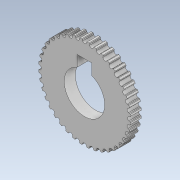
# Autodesk Inventor part: 2GT_40T
Saved by Autodesk Inventor 2022 (Build 260153000, 153)
## iProperties
Created: 2023-05-04
Part Number: 2GT_40T
Material: 一般
Document SubType Name: Modeling
Designer: Johnny Jou
Density: 1 g/cm^3
Appearance: 預設
Author: Johnny Jou
Autodesk Inventor part; units mm, degrees
ref_plane "YZ Plane" through (0, 0, 0) normal (1, 0, 0) x (0, 1, 0)
ref_plane "XZ Plane" through (0, 0, 0) normal (0, 1, 0) x (-1, 0, 0)
ref_plane "XY Plane" through (0, 0, 0) normal (0, 0, 1) x (1, 0, 0)
sketch "草圖1" plane through (0, 0, 0) normal (0, 0, 1) x (1, 0, 0)
  arc A0 (1.3466, 12.2657) -> (1.2112, 12.4161) centre (1.1966, 12.2668) ccw
  arc A1 (1.2112, 12.4161) -> (0.746, 12.4527) centre (0, 0) ccw
  arc A2 (0.746, 12.4527) -> (0.5887, 12.3254) centre (0.7371, 12.3029) ccw
  arc A3 (0.4989, 12.0368) -> (0.5887, 12.3254) centre (-0.4, 12.475) ccw
  arc A4 (-0.4989, 12.0368) -> (0.4989, 12.0368) centre (0, 12.28) ccw
  arc A5 (-0.5887, 12.3254) -> (-0.4989, 12.0368) centre (0.4, 12.475) ccw
  arc A6 (-0.5887, 12.3254) -> (-0.746, 12.4527) centre (-0.7371, 12.3029) ccw
  arc A7 (-0.746, 12.4527) -> (-1.2112, 12.4161) centre (0, 0) ccw
  arc A8 (-1.2112, 12.4161) -> (-1.3466, 12.2657) centre (-1.1966, 12.2668) ccw
  arc A9 (-1.3902, 11.9666) -> (-1.3466, 12.2657) centre (-2.3466, 12.2588) ccw
  arc A10 (-2.3757, 11.8106) -> (-1.3902, 11.9666) centre (-1.921, 12.1288) ccw
  arc A11 (-2.5096, 12.0815) -> (-2.3757, 11.8106) centre (-1.5564, 12.384) ccw
  arc A12 (-2.5096, 12.0815) -> (-2.6849, 12.1827) centre (-2.6526, 12.0362) ccw
  arc A13 (-2.6849, 12.1827) -> (-3.1386, 12.0737) centre (0, 0) ccw
  arc A14 (-3.1386, 12.0737) -> (-3.2488, 11.9041) centre (-3.1008, 11.9286) ccw
  arc A15 (-3.2451, 11.6018) -> (-3.2488, 11.9041) centre (-4.2354, 11.7408) ccw
  arc A16 (-4.194, 11.2935) -> (-3.2451, 11.6018) centre (-3.7947, 11.679) ccw
  arc A17 (-4.3687, 11.5402) -> (-4.194, 11.2935) centre (-3.4746, 11.988) ccw
  arc A18 (-4.3687, 11.5402) -> (-4.5576, 11.6127) centre (-4.5028, 11.473) ccw
  arc A19 (-4.5576, 11.6127) -> (-4.9887, 11.4341) centre (0, 0) ccw
  arc A20 (-4.9887, 11.4341) -> (-5.071, 11.2493) centre (-4.9287, 11.2966) ccw
  arc A21 (-5.0201, 10.9514) -> (-5.071, 11.2493) centre (-6.0199, 10.9337) ccw
  arc A22 (-5.9091, 10.4984) -> (-5.0201, 10.9514) centre (-5.575, 10.9416) ccw
  arc A23 (-6.1202, 10.7147) -> (-5.9091, 10.4984) centre (-5.3071, 11.2969) ccw
  arc A24 (-6.1202, 10.7147) -> (-6.3181, 10.7567) centre (-6.2421, 10.6274) ccw
  arc A25 (-6.3181, 10.7567) -> (-6.7159, 10.5129) centre (0, 0) ccw
  arc A26 (-6.7159, 10.5129) -> (-6.7684, 10.3175) centre (-6.6352, 10.3865) ccw
  arc A27 (-6.6715, 10.0312) -> (-6.7684, 10.3175) centre (-7.6562, 9.8574) ccw
  arc A28 (-7.4787, 9.4447) -> (-6.6715, 10.0312) centre (-7.218, 9.9347) ccw
  arc A29 (-7.721, 9.6254) -> (-7.4787, 9.4447) centre (-7.009, 10.3276) ccw
  arc A30 (-7.721, 9.6254) -> (-7.923, 9.6359) centre (-7.8278, 9.5201) ccw
  arc A31 (-7.923, 9.6359) -> (-8.2778, 9.3329) centre (0, 0) ccw
  arc A32 (-8.2778, 9.3329) -> (-8.2991, 9.1317) centre (-8.1783, 9.2207) ccw
  arc A33 (-8.1585, 8.8641) -> (-8.2991, 9.1317) centre (-9.104, 8.5383) ccw
  arc A34 (-8.8641, 8.1585) -> (-8.1585, 8.8641) centre (-8.6833, 8.6833) ccw
  arc A35 (-9.1317, 8.2991) -> (-8.8641, 8.1585) centre (-8.5383, 9.104) ccw
  arc A36 (-9.1317, 8.2991) -> (-9.3329, 8.2778) centre (-9.2207, 8.1783) ccw
  arc A37 (-9.3329, 8.2778) -> (-9.6359, 7.923) centre (0, 0) ccw
  arc A38 (-9.6359, 7.923) -> (-9.6254, 7.721) centre (-9.5201, 7.8278) ccw
  arc A39 (-9.4447, 7.4787) -> (-9.6254, 7.721) centre (-10.3276, 7.009) ccw
  arc A40 (-10.0312, 6.6715) -> (-9.4447, 7.4787) centre (-9.9347, 7.218) ccw
  arc A41 (-10.3175, 6.7684) -> (-10.0312, 6.6715) centre (-9.8574, 7.6562) ccw
  arc A42 (-10.3175, 6.7684) -> (-10.5129, 6.7159) centre (-10.3865, 6.6352) ccw
  arc A43 (-10.5129, 6.7159) -> (-10.7567, 6.3181) centre (0, 0) ccw
  arc A44 (-10.7567, 6.3181) -> (-10.7147, 6.1202) centre (-10.6274, 6.2421) ccw
  arc A45 (-10.4984, 5.9091) -> (-10.7147, 6.1202) centre (-11.2969, 5.3071) ccw
  arc A46 (-10.9514, 5.0201) -> (-10.4984, 5.9091) centre (-10.9416, 5.575) ccw
  arc A47 (-11.2493, 5.071) -> (-10.9514, 5.0201) centre (-10.9337, 6.0199) ccw
  arc A48 (-11.2493, 5.071) -> (-11.4341, 4.9887) centre (-11.2966, 4.9287) ccw
  arc A49 (-11.4341, 4.9887) -> (-11.6127, 4.5576) centre (0, 0) ccw
  arc A50 (-11.6127, 4.5576) -> (-11.5402, 4.3687) centre (-11.473, 4.5028) ccw
  arc A51 (-11.2935, 4.194) -> (-11.5402, 4.3687) centre (-11.988, 3.4746) ccw
  arc A52 (-11.6018, 3.2451) -> (-11.2935, 4.194) centre (-11.679, 3.7947) ccw
  arc A53 (-11.9041, 3.2488) -> (-11.6018, 3.2451) centre (-11.7408, 4.2354) ccw
  arc A54 (-11.9041, 3.2488) -> (-12.0737, 3.1386) centre (-11.9286, 3.1008) ccw
  arc A55 (-12.0737, 3.1386) -> (-12.1827, 2.6849) centre (0, 0) ccw
  arc A56 (-12.1827, 2.6849) -> (-12.0815, 2.5096) centre (-12.0362, 2.6526) ccw
  arc A57 (-11.8106, 2.3757) -> (-12.0815, 2.5096) centre (-12.384, 1.5564) ccw
  arc A58 (-11.9666, 1.3902) -> (-11.8106, 2.3757) centre (-12.1288, 1.921) ccw
  arc A59 (-12.2657, 1.3466) -> (-11.9666, 1.3902) centre (-12.2588, 2.3466) ccw
  arc A60 (-12.2657, 1.3466) -> (-12.4161, 1.2112) centre (-12.2668, 1.1966) ccw
  arc A61 (-12.4161, 1.2112) -> (-12.4527, 0.746) centre (0, 0) ccw
  arc A62 (-12.4527, 0.746) -> (-12.3254, 0.5887) centre (-12.3029, 0.7371) ccw
  arc A63 (-12.0368, 0.4989) -> (-12.3254, 0.5887) centre (-12.475, -0.4) ccw
  arc A64 (-12.0368, -0.4989) -> (-12.0368, 0.4989) centre (-12.28, 0) ccw
  arc A65 (-12.3254, -0.5887) -> (-12.0368, -0.4989) centre (-12.475, 0.4) ccw
  arc A66 (-12.3254, -0.5887) -> (-12.4527, -0.746) centre (-12.3029, -0.7371) ccw
  arc A67 (-12.4527, -0.746) -> (-12.4161, -1.2112) centre (0, 0) ccw
  arc A68 (-12.4161, -1.2112) -> (-12.2657, -1.3466) centre (-12.2668, -1.1966) ccw
  arc A69 (-11.9666, -1.3902) -> (-12.2657, -1.3466) centre (-12.2588, -2.3466) ccw
  arc A70 (-11.8106, -2.3757) -> (-11.9666, -1.3902) centre (-12.1288, -1.921) ccw
  arc A71 (-12.0815, -2.5096) -> (-11.8106, -2.3757) centre (-12.384, -1.5564) ccw
  arc A72 (-12.0815, -2.5096) -> (-12.1827, -2.6849) centre (-12.0362, -2.6526) ccw
  arc A73 (-12.1827, -2.6849) -> (-12.0737, -3.1386) centre (0, 0) ccw
  arc A74 (-12.0737, -3.1386) -> (-11.9041, -3.2488) centre (-11.9286, -3.1008) ccw
  arc A75 (-11.6018, -3.2451) -> (-11.9041, -3.2488) centre (-11.7408, -4.2354) ccw
  arc A76 (-11.2935, -4.194) -> (-11.6018, -3.2451) centre (-11.679, -3.7947) ccw
  arc A77 (-11.5402, -4.3687) -> (-11.2935, -4.194) centre (-11.988, -3.4746) ccw
  arc A78 (-11.5402, -4.3687) -> (-11.6127, -4.5576) centre (-11.473, -4.5028) ccw
  arc A79 (-11.6127, -4.5576) -> (-11.4341, -4.9887) centre (0, 0) ccw
  arc A80 (-11.4341, -4.9887) -> (-11.2493, -5.071) centre (-11.2966, -4.9287) ccw
  arc A81 (-10.9514, -5.0201) -> (-11.2493, -5.071) centre (-10.9337, -6.0199) ccw
  arc A82 (-10.4984, -5.9091) -> (-10.9514, -5.0201) centre (-10.9416, -5.575) ccw
  arc A83 (-10.7147, -6.1202) -> (-10.4984, -5.9091) centre (-11.2969, -5.3071) ccw
  arc A84 (-10.7147, -6.1202) -> (-10.7567, -6.3181) centre (-10.6274, -6.2421) ccw
  arc A85 (-10.7567, -6.3181) -> (-10.5129, -6.7159) centre (0, 0) ccw
  arc A86 (-10.5129, -6.7159) -> (-10.3175, -6.7684) centre (-10.3865, -6.6352) ccw
  arc A87 (-10.0312, -6.6715) -> (-10.3175, -6.7684) centre (-9.8574, -7.6562) ccw
  arc A88 (-9.4447, -7.4787) -> (-10.0312, -6.6715) centre (-9.9347, -7.218) ccw
  arc A89 (-9.6254, -7.721) -> (-9.4447, -7.4787) centre (-10.3276, -7.009) ccw
  arc A90 (-9.6254, -7.721) -> (-9.6359, -7.923) centre (-9.5201, -7.8278) ccw
  arc A91 (-9.6359, -7.923) -> (-9.3329, -8.2778) centre (0, 0) ccw
  arc A92 (-9.3329, -8.2778) -> (-9.1317, -8.2991) centre (-9.2207, -8.1783) ccw
  arc A93 (-8.8641, -8.1585) -> (-9.1317, -8.2991) centre (-8.5383, -9.104) ccw
  arc A94 (-8.1585, -8.8641) -> (-8.8641, -8.1585) centre (-8.6833, -8.6833) ccw
  arc A95 (-8.2991, -9.1317) -> (-8.1585, -8.8641) centre (-9.104, -8.5383) ccw
  arc A96 (-8.2991, -9.1317) -> (-8.2778, -9.3329) centre (-8.1783, -9.2207) ccw
  arc A97 (-8.2778, -9.3329) -> (-7.923, -9.6359) centre (0, 0) ccw
  arc A98 (-7.923, -9.6359) -> (-7.721, -9.6254) centre (-7.8278, -9.5201) ccw
  arc A99 (-7.4787, -9.4447) -> (-7.721, -9.6254) centre (-7.009, -10.3276) ccw
  arc A100 (-6.6715, -10.0312) -> (-7.4787, -9.4447) centre (-7.218, -9.9347) ccw
  arc A101 (-6.7684, -10.3175) -> (-6.6715, -10.0312) centre (-7.6562, -9.8574) ccw
  arc A102 (-6.7684, -10.3175) -> (-6.7159, -10.5129) centre (-6.6352, -10.3865) ccw
  arc A103 (-6.7159, -10.5129) -> (-6.3181, -10.7567) centre (0, 0) ccw
  arc A104 (-6.3181, -10.7567) -> (-6.1202, -10.7147) centre (-6.2421, -10.6274) ccw
  arc A105 (-5.9091, -10.4984) -> (-6.1202, -10.7147) centre (-5.3071, -11.2969) ccw
  arc A106 (-5.0201, -10.9514) -> (-5.9091, -10.4984) centre (-5.575, -10.9416) ccw
  arc A107 (-5.071, -11.2493) -> (-5.0201, -10.9514) centre (-6.0199, -10.9337) ccw
  arc A108 (-5.071, -11.2493) -> (-4.9887, -11.4341) centre (-4.9287, -11.2966) ccw
  arc A109 (-4.9887, -11.4341) -> (-4.5576, -11.6127) centre (0, 0) ccw
  arc A110 (-4.5576, -11.6127) -> (-4.3687, -11.5402) centre (-4.5028, -11.473) ccw
  arc A111 (-4.194, -11.2935) -> (-4.3687, -11.5402) centre (-3.4746, -11.988) ccw
  arc A112 (-3.2451, -11.6018) -> (-4.194, -11.2935) centre (-3.7947, -11.679) ccw
  arc A113 (-3.2488, -11.9041) -> (-3.2451, -11.6018) centre (-4.2354, -11.7408) ccw
  arc A114 (-3.2488, -11.9041) -> (-3.1386, -12.0737) centre (-3.1008, -11.9286) ccw
  arc A115 (-3.1386, -12.0737) -> (-2.6849, -12.1827) centre (0, 0) ccw
  arc A116 (-2.6849, -12.1827) -> (-2.5096, -12.0815) centre (-2.6526, -12.0362) ccw
  arc A117 (-2.3757, -11.8106) -> (-2.5096, -12.0815) centre (-1.5564, -12.384) ccw
  arc A118 (-1.3902, -11.9666) -> (-2.3757, -11.8106) centre (-1.921, -12.1288) ccw
  arc A119 (-1.3466, -12.2657) -> (-1.3902, -11.9666) centre (-2.3466, -12.2588) ccw
  arc A120 (-1.3466, -12.2657) -> (-1.2112, -12.4161) centre (-1.1966, -12.2668) ccw
  arc A121 (-1.2112, -12.4161) -> (-0.746, -12.4527) centre (0, 0) ccw
  arc A122 (-0.746, -12.4527) -> (-0.5887, -12.3254) centre (-0.7371, -12.3029) ccw
  arc A123 (-0.4989, -12.0368) -> (-0.5887, -12.3254) centre (0.4, -12.475) ccw
  arc A124 (0.4989, -12.0368) -> (-0.4989, -12.0368) centre (0, -12.28) ccw
  arc A125 (0.5887, -12.3254) -> (0.4989, -12.0368) centre (-0.4, -12.475) ccw
  arc A126 (0.5887, -12.3254) -> (0.746, -12.4527) centre (0.7371, -12.3029) ccw
  arc A127 (0.746, -12.4527) -> (1.2112, -12.4161) centre (0, 0) ccw
  arc A128 (1.2112, -12.4161) -> (1.3466, -12.2657) centre (1.1966, -12.2668) ccw
  arc A129 (1.3902, -11.9666) -> (1.3466, -12.2657) centre (2.3466, -12.2588) ccw
  arc A130 (2.3757, -11.8106) -> (1.3902, -11.9666) centre (1.921, -12.1288) ccw
  arc A131 (2.5096, -12.0815) -> (2.3757, -11.8106) centre (1.5564, -12.384) ccw
  arc A132 (2.5096, -12.0815) -> (2.6849, -12.1827) centre (2.6526, -12.0362) ccw
  arc A133 (2.6849, -12.1827) -> (3.1386, -12.0737) centre (0, 0) ccw
  arc A134 (3.1386, -12.0737) -> (3.2488, -11.9041) centre (3.1008, -11.9286) ccw
  arc A135 (3.2451, -11.6018) -> (3.2488, -11.9041) centre (4.2354, -11.7408) ccw
  arc A136 (4.194, -11.2935) -> (3.2451, -11.6018) centre (3.7947, -11.679) ccw
  arc A137 (4.3687, -11.5402) -> (4.194, -11.2935) centre (3.4746, -11.988) ccw
  arc A138 (4.3687, -11.5402) -> (4.5576, -11.6127) centre (4.5028, -11.473) ccw
  arc A139 (4.5576, -11.6127) -> (4.9887, -11.4341) centre (0, 0) ccw
  arc A140 (4.9887, -11.4341) -> (5.071, -11.2493) centre (4.9287, -11.2966) ccw
  arc A141 (5.0201, -10.9514) -> (5.071, -11.2493) centre (6.0199, -10.9337) ccw
  arc A142 (5.9091, -10.4984) -> (5.0201, -10.9514) centre (5.575, -10.9416) ccw
  arc A143 (6.1202, -10.7147) -> (5.9091, -10.4984) centre (5.3071, -11.2969) ccw
  arc A144 (6.1202, -10.7147) -> (6.3181, -10.7567) centre (6.2421, -10.6274) ccw
  arc A145 (6.3181, -10.7567) -> (6.7159, -10.5129) centre (0, 0) ccw
  arc A146 (6.7159, -10.5129) -> (6.7684, -10.3175) centre (6.6352, -10.3865) ccw
  arc A147 (6.6715, -10.0312) -> (6.7684, -10.3175) centre (7.6562, -9.8574) ccw
  arc A148 (7.4787, -9.4447) -> (6.6715, -10.0312) centre (7.218, -9.9347) ccw
  arc A149 (7.721, -9.6254) -> (7.4787, -9.4447) centre (7.009, -10.3276) ccw
  arc A150 (7.721, -9.6254) -> (7.923, -9.6359) centre (7.8278, -9.5201) ccw
  arc A151 (7.923, -9.6359) -> (8.2778, -9.3329) centre (0, 0) ccw
  arc A152 (8.2778, -9.3329) -> (8.2991, -9.1317) centre (8.1783, -9.2207) ccw
  arc A153 (8.1585, -8.8641) -> (8.2991, -9.1317) centre (9.104, -8.5383) ccw
  arc A154 (8.8641, -8.1585) -> (8.1585, -8.8641) centre (8.6833, -8.6833) ccw
  arc A155 (9.1317, -8.2991) -> (8.8641, -8.1585) centre (8.5383, -9.104) ccw
  arc A156 (9.1317, -8.2991) -> (9.3329, -8.2778) centre (9.2207, -8.1783) ccw
  arc A157 (9.3329, -8.2778) -> (9.6359, -7.923) centre (0, 0) ccw
  arc A158 (9.6359, -7.923) -> (9.6254, -7.721) centre (9.5201, -7.8278) ccw
  arc A159 (9.4447, -7.4787) -> (9.6254, -7.721) centre (10.3276, -7.009) ccw
  arc A160 (10.0312, -6.6715) -> (9.4447, -7.4787) centre (9.9347, -7.218) ccw
  arc A161 (10.3175, -6.7684) -> (10.0312, -6.6715) centre (9.8574, -7.6562) ccw
  arc A162 (10.3175, -6.7684) -> (10.5129, -6.7159) centre (10.3865, -6.6352) ccw
  arc A163 (10.5129, -6.7159) -> (10.7567, -6.3181) centre (0, 0) ccw
  arc A164 (10.7567, -6.3181) -> (10.7147, -6.1202) centre (10.6274, -6.2421) ccw
  arc A165 (10.4984, -5.9091) -> (10.7147, -6.1202) centre (11.2969, -5.3071) ccw
  arc A166 (10.9514, -5.0201) -> (10.4984, -5.9091) centre (10.9416, -5.575) ccw
  arc A167 (11.2493, -5.071) -> (10.9514, -5.0201) centre (10.9337, -6.0199) ccw
  arc A168 (11.2493, -5.071) -> (11.4341, -4.9887) centre (11.2966, -4.9287) ccw
  arc A169 (11.4341, -4.9887) -> (11.6127, -4.5576) centre (0, 0) ccw
  arc A170 (11.6127, -4.5576) -> (11.5402, -4.3687) centre (11.473, -4.5028) ccw
  arc A171 (11.2935, -4.194) -> (11.5402, -4.3687) centre (11.988, -3.4746) ccw
  arc A172 (11.6018, -3.2451) -> (11.2935, -4.194) centre (11.679, -3.7947) ccw
  arc A173 (11.9041, -3.2488) -> (11.6018, -3.2451) centre (11.7408, -4.2354) ccw
  arc A174 (11.9041, -3.2488) -> (12.0737, -3.1386) centre (11.9286, -3.1008) ccw
  arc A175 (12.0737, -3.1386) -> (12.1827, -2.6849) centre (0, 0) ccw
  arc A176 (12.1827, -2.6849) -> (12.0815, -2.5096) centre (12.0362, -2.6526) ccw
  arc A177 (11.8106, -2.3757) -> (12.0815, -2.5096) centre (12.384, -1.5564) ccw
  arc A178 (11.9666, -1.3902) -> (11.8106, -2.3757) centre (12.1288, -1.921) ccw
  arc A179 (12.2657, -1.3466) -> (11.9666, -1.3902) centre (12.2588, -2.3466) ccw
  arc A180 (12.2657, -1.3466) -> (12.4161, -1.2112) centre (12.2668, -1.1966) ccw
  arc A181 (12.4161, -1.2112) -> (12.4527, -0.746) centre (0, 0) ccw
  arc A182 (12.4527, -0.746) -> (12.3254, -0.5887) centre (12.3029, -0.7371) ccw
  arc A183 (12.0368, -0.4989) -> (12.3254, -0.5887) centre (12.475, 0.4) ccw
  arc A184 (12.0368, 0.4989) -> (12.0368, -0.4989) centre (12.28, 0) ccw
  arc A185 (12.3254, 0.5887) -> (12.0368, 0.4989) centre (12.475, -0.4) ccw
  arc A186 (12.3254, 0.5887) -> (12.4527, 0.746) centre (12.3029, 0.7371) ccw
  arc A187 (12.4527, 0.746) -> (12.4161, 1.2112) centre (0, 0) ccw
  arc A188 (12.4161, 1.2112) -> (12.2657, 1.3466) centre (12.2668, 1.1966) ccw
  arc A189 (11.9666, 1.3902) -> (12.2657, 1.3466) centre (12.2588, 2.3466) ccw
  arc A190 (11.8106, 2.3757) -> (11.9666, 1.3902) centre (12.1288, 1.921) ccw
  arc A191 (12.0815, 2.5096) -> (11.8106, 2.3757) centre (12.384, 1.5564) ccw
  arc A192 (12.0815, 2.5096) -> (12.1827, 2.6849) centre (12.0362, 2.6526) ccw
  arc A193 (12.1827, 2.6849) -> (12.0737, 3.1386) centre (0, 0) ccw
  arc A194 (12.0737, 3.1386) -> (11.9041, 3.2488) centre (11.9286, 3.1008) ccw
  arc A195 (11.6018, 3.2451) -> (11.9041, 3.2488) centre (11.7408, 4.2354) ccw
  arc A196 (11.2935, 4.194) -> (11.6018, 3.2451) centre (11.679, 3.7947) ccw
  arc A197 (11.5402, 4.3687) -> (11.2935, 4.194) centre (11.988, 3.4746) ccw
  arc A198 (11.5402, 4.3687) -> (11.6127, 4.5576) centre (11.473, 4.5028) ccw
  arc A199 (11.6127, 4.5576) -> (11.4341, 4.9887) centre (0, 0) ccw
  arc A200 (11.4341, 4.9887) -> (11.2493, 5.071) centre (11.2966, 4.9287) ccw
  arc A201 (10.9514, 5.0201) -> (11.2493, 5.071) centre (10.9337, 6.0199) ccw
  arc A202 (10.4984, 5.9091) -> (10.9514, 5.0201) centre (10.9416, 5.575) ccw
  arc A203 (10.7147, 6.1202) -> (10.4984, 5.9091) centre (11.2969, 5.3071) ccw
  arc A204 (10.7147, 6.1202) -> (10.7567, 6.3181) centre (10.6274, 6.2421) ccw
  arc A205 (10.7567, 6.3181) -> (10.5129, 6.7159) centre (0, 0) ccw
  arc A206 (10.5129, 6.7159) -> (10.3175, 6.7684) centre (10.3865, 6.6352) ccw
  arc A207 (10.0312, 6.6715) -> (10.3175, 6.7684) centre (9.8574, 7.6562) ccw
  arc A208 (9.4447, 7.4787) -> (10.0312, 6.6715) centre (9.9347, 7.218) ccw
  arc A209 (9.6254, 7.721) -> (9.4447, 7.4787) centre (10.3276, 7.009) ccw
  arc A210 (9.6254, 7.721) -> (9.6359, 7.923) centre (9.5201, 7.8278) ccw
  arc A211 (9.6359, 7.923) -> (9.3329, 8.2778) centre (0, 0) ccw
  arc A212 (9.3329, 8.2778) -> (9.1317, 8.2991) centre (9.2207, 8.1783) ccw
  arc A213 (8.8641, 8.1585) -> (9.1317, 8.2991) centre (8.5383, 9.104) ccw
  arc A214 (8.1585, 8.8641) -> (8.8641, 8.1585) centre (8.6833, 8.6833) ccw
  arc A215 (8.2991, 9.1317) -> (8.1585, 8.8641) centre (9.104, 8.5383) ccw
  arc A216 (8.2991, 9.1317) -> (8.2778, 9.3329) centre (8.1783, 9.2207) ccw
  arc A217 (8.2778, 9.3329) -> (7.923, 9.6359) centre (0, 0) ccw
  arc A218 (7.923, 9.6359) -> (7.721, 9.6254) centre (7.8278, 9.5201) ccw
  arc A219 (7.4787, 9.4447) -> (7.721, 9.6254) centre (7.009, 10.3276) ccw
  arc A220 (6.6715, 10.0312) -> (7.4787, 9.4447) centre (7.218, 9.9347) ccw
  arc A221 (6.7684, 10.3175) -> (6.6715, 10.0312) centre (7.6562, 9.8574) ccw
  arc A222 (6.7684, 10.3175) -> (6.7159, 10.5129) centre (6.6352, 10.3865) ccw
  arc A223 (6.7159, 10.5129) -> (6.3181, 10.7567) centre (0, 0) ccw
  arc A224 (6.3181, 10.7567) -> (6.1202, 10.7147) centre (6.2421, 10.6274) ccw
  arc A225 (5.9091, 10.4984) -> (6.1202, 10.7147) centre (5.3071, 11.2969) ccw
  arc A226 (5.0201, 10.9514) -> (5.9091, 10.4984) centre (5.575, 10.9416) ccw
  arc A227 (5.071, 11.2493) -> (5.0201, 10.9514) centre (6.0199, 10.9337) ccw
  arc A228 (5.071, 11.2493) -> (4.9887, 11.4341) centre (4.9287, 11.2966) ccw
  arc A229 (4.9887, 11.4341) -> (4.5576, 11.6127) centre (0, 0) ccw
  arc A230 (4.5576, 11.6127) -> (4.3687, 11.5402) centre (4.5028, 11.473) ccw
  arc A231 (4.194, 11.2935) -> (4.3687, 11.5402) centre (3.4746, 11.988) ccw
  arc A232 (3.2451, 11.6018) -> (4.194, 11.2935) centre (3.7947, 11.679) ccw
  arc A233 (3.2488, 11.9041) -> (3.2451, 11.6018) centre (4.2354, 11.7408) ccw
  arc A234 (3.2488, 11.9041) -> (3.1386, 12.0737) centre (3.1008, 11.9286) ccw
  arc A235 (3.1386, 12.0737) -> (2.6849, 12.1827) centre (0, 0) ccw
  arc A236 (2.6849, 12.1827) -> (2.5096, 12.0815) centre (2.6526, 12.0362) ccw
  arc A237 (2.3757, 11.8106) -> (2.5096, 12.0815) centre (1.5564, 12.384) ccw
  arc A238 (1.3902, 11.9666) -> (2.3757, 11.8106) centre (1.921, 12.1288) ccw
  arc A239 (1.3466, 12.2657) -> (1.3902, 11.9666) centre (2.3466, 12.2588) ccw
  circle A240 centre (0, 0) radius 5.5
  line L0 (-2, 8.1235) -> (2, 8.1235)
  line L1 (2, 8.1235) -> (2, 5.1235)
  line L2 (2, 5.1235) -> (-2, 5.1235)
  line L3 (-2, 5.1235) -> (-2, 8.1235)
  point P0 (0, 0)
  point P1 (0, 0)
  dimension "d0" = 11
  dimension "d1" = 4
  dimension "d2" = 3
  constraints: 482 point on circle, 241 centre point, 8 end point, 2 parallel, 1 coincident, 1 horizontal, 1 perpendicular, 680 other
  measures "d0" diameter of A240
  measures "d1" distance of L0.start L0.end
  measures "d2" distance of L0.end L1.end
extrude "擠出1" add sketch "草圖1" along normal blind 3
